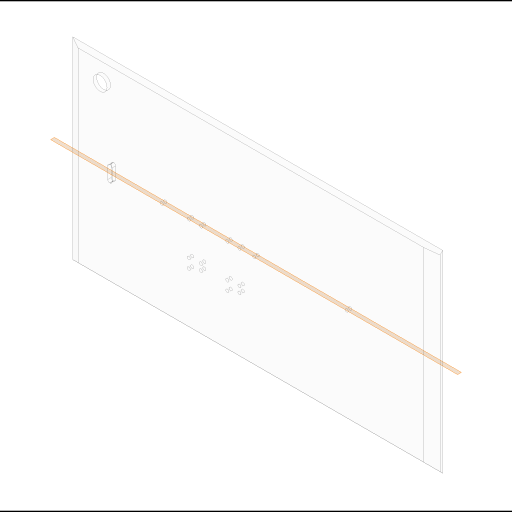
# Autodesk Inventor part: Wind Tunnel Test Section Bottom
Saved by Autodesk Inventor 2023 (Build 270158000, 158)
## iProperties
Created: 2022-03-05
Part Number: Wind Tunnel Test Section Bottom
Material: Polycarbonate, Clear
Document SubType Name: Modeling
Designer: kamer
Density: 1.2 g/cm^3
Appearance: Polycarbonate - Clear
Author: kamer
Autodesk Inventor part; units mm, degrees
ref_plane "YZ Plane" through (0, 0, 0) normal (1, 0, 0) x (0, 1, 0)
ref_plane "XY Plane" through (0, 0, 0) normal (0, 0, 1) x (1, 0, 0)
sketch "Sketch1" plane through (0, 0, 0) normal (0, 0, 1) x (1, 0, 0)
  line L0 (0, 0) -> (609.6, 0)
  line L1 (609.6, 0) -> (609.6, 317.881)
  line L2 (609.6, 317.881) -> (0, 317.881)
  line L3 (0, 317.881) -> (0, 0)
  dimension "d0" = 609.6
  dimension "d1" = 317.881
  constraints: 8 end point, 2 parallel, 1 horizontal, 1 perpendicular
  measures "d0" distance of L1.end L2.end
  measures "d1" distance of L0.end L1.end
extrude "Extrusion1" add sketch "Sketch1" along normal blind 5.7658
sketch "Sketch2" plane through (0, 317.881, 0) normal (0, 1, 0) x (1, 0, 0)
  line L0 (609.6, 0) -> (0, 0) projected
  line L1 (0, 0) -> (0, -5.7658) projected
  line L2 (609.6, -5.7658) -> (0, -5.7658) projected
  line L3 (609.6, 0) -> (609.6, -5.7658) projected
  line L4 (0, 0) -> (609.6, 0) projected
  line L5 (0, 0) -> (14.4594, -5.7658)
  line L6 (0, -5.7658) -> (609.6, -5.7658) projected
  line L7 (14.4594, -5.7658) -> (14.4594, 0)
  line L8 (14.4594, -5.7658) -> (20.2252, -5.7658) construction
  dimension "d4" = 21.74
  dimension "d5" = 90
  constraints: 6 end point, 2 point on line, 1 horizontal, 1 perpendicular
  measures "d4" angle of L5 L0
  measures "d5" angle of L8 L7
extrude "Extrusion2" cut sketch "Sketch2" against normal through all contours L5 L2 L1
sketch "Sketch3" plane through (609.6, 0, 0) normal (1, 0, 0) x (0, 0, -1)
  line L0 (0, 0) -> (0, 317.881) projected
  line L1 (0, 317.881) -> (-5.7658, 317.881) projected
  line L2 (-5.7658, 0) -> (-5.7658, 317.881) projected
  line L3 (0, 0) -> (-5.7658, 0) projected
  line L4 (0, 0) -> (-5.7658, 0) projected
  line L5 (0, 0) -> (-5.7658, 5.7658)
  line L6 (-5.7658, 0) -> (-5.7658, 317.881) projected
  line L7 (0, 0) -> (8.1541, 0) construction
  line L8 (0, 317.881) -> (-5.7658, 317.881) projected
  line L9 (0, 317.881) -> (-5.7658, 312.1152)
  line L10 (0, 317.881) -> (8.1541, 317.881) construction
  dimension "d8" = 135
  dimension "d9" = 135
  constraints: 8 end point, 2 equal length, 2 horizontal, 2 point on line
  measures "d8" angle of L7 L5
  measures "d9" angle of L9 L10
extrude "Extrusion3" cut sketch "Sketch3" against normal through all contours L3 L2 L5 | L9 L2 L1
ref_plane "Center Plane" through (0, 158.9405, 0) normal (0, 1, 0) x (-1, 0, 0)
sketch "Sketch4" plane through (0, 158.9405, 0) normal (0, 1, 0) x (-1, 0, 0)
  line L0 (-14.4594, 5.7658) -> (0, 0) projected
  line L1 (-609.6, 5.7658) -> (-14.4594, 5.7658) projected
  line L2 (-609.6, 0) -> (-609.6, 5.7658) projected
  line L3 (-609.6, 0) -> (0, 0) projected
  line L4 (-609.6, 5.7658) -> (-584.2, 5.7658) construction
  line L5 (-584.2, 5.7658) -> (-609.6, 4.4413)
  point P0 (0, 0)
  dimension "d13" = 25.4
  dimension "d14" = 2.985
  constraints: 4 end point, 2 point on line
  measures "d13" distance of L1.start L4.end
  measures "d14" angle of L4 L5
extrude "Extrusion4" cut sketch "Sketch4" against normal through all both and the other way through all contours L5 L2 L1
sketch "Sketch5" plane through (0, 0, 5.7658) normal (0, 0, 1) x (1, 0, 0)
  circle A0 centre (196.85, 158.9278) radius 2.5019
  line L0 (0, 317.881) -> (0, 0) projected
  line L1 (609.6, 317.881) -> (0, 317.881) projected
  circle A1 centre (260.35, 158.9405) radius 2.5019
  circle A2 centre (196.85, 103.5558) radius 2.5019
  circle A3 centre (260.35, 103.5685) radius 2.5019
  circle A4 centre (196.85, 88.3158) radius 2.5019
  circle A5 centre (260.35, 88.3285) radius 2.5019
  circle A6 centre (152.4, 158.9405) radius 2.5019
  circle A7 centre (304.8, 158.9405) radius 2.5019
  circle A8 centre (457.2, 158.9405) radius 2.5019
  line L2 (66.675, 145.7528) -> (67.325, 145.7528)
  line L3 (70.5, 148.9278) -> (70.5, 168.9278)
  line L4 (67.325, 172.1028) -> (66.675, 172.1028)
  line L5 (63.5, 168.9278) -> (63.5, 148.9278)
  line L6 (63.5, 145.7528) -> (70.5, 172.1028) construction
  line L7 (70.5, 145.7528) -> (63.5, 172.1028) construction
  arc A9 (70.5, 168.9278) -> (67.325, 172.1028) centre (67.325, 168.9278) ccw
  arc A10 (66.675, 172.1028) -> (63.5, 168.9278) centre (66.675, 168.9278) ccw
  arc A11 (63.5, 148.9278) -> (66.675, 145.7528) centre (66.675, 148.9278) ccw
  arc A12 (67.325, 145.7528) -> (70.5, 148.9278) centre (67.325, 148.9278) ccw
  point P0 (67, 158.9278)
  dimension "d17" = 196.85
  dimension "d18" = 158.9532
  dimension "d19" = 5.0038
  dimension "d20" = 63.5
  dimension "d21" = 5.0038
  dimension "d22" = 55.372
  dimension "d23" = 55.372
  dimension "d24" = 196.85
  dimension "d25" = 63.5
  dimension "d26" = 158.9405
  dimension "d27" = 5.0038
  dimension "d28" = 5.0038
  dimension "d29" = 15.24
  dimension "d30" = 15.24
  dimension "d31" = 5.0038
  dimension "d32" = 5.0038
  dimension "d33" = 63.5
  dimension "d34" = 196.85
  dimension "d35" = 152.4
  dimension "d36" = 5.0038
  dimension "d37" = 158.9405
  dimension "d38" = 304.8
  dimension "d39" = 5.0038
  dimension "d40" = 158.9405
  dimension "d41" = 457.2
  dimension "d42" = 158.9405
  dimension "d43" = 5.0038
  dimension "d44" = 3.175
  dimension "d45" = 7
  dimension "d46" = 20
  dimension "d47" = 158.9532
  dimension "d48" = 63.5
  constraints: 13 centre point, 12 end point, 8 point on circle, 8 point on line, 8 tangent, 3 equal radius, 2 midpoint, 2 parallel, 1 horizontal, 1 perpendicular
  measures "d17" distance from line of A0.centre L0
  measures "d18" distance from line of A0.centre L1
  measures "d19" diameter of A0
  measures "d20" distance of A1.centre A0.centre
  measures "d21" diameter of A1
  measures "d22" distance of A0.centre A2.centre
  measures "d23" distance of A3.centre A1.centre
  measures "d24" distance from line of L0 A2.centre
  measures "d25" distance of A2.centre A3.centre
  measures "d26" distance from line of L1 A1.centre
  measures "d27" diameter of A2
  measures "d28" diameter of A3
  measures "d29" distance of A4.centre A2.centre
  measures "d30" distance of A5.centre A3.centre
  measures "d31" diameter of A4
  measures "d32" diameter of A5
  measures "d33" distance of A4.centre A5.centre
  measures "d34" distance from line of L0 A4.centre
  measures "d35" distance from line of L0 A6.centre
  measures "d36" diameter of A6
  measures "d37" distance from line of A6.centre L1
  measures "d38" distance from line of L0 A7.centre
  measures "d39" diameter of A7
  measures "d40" distance from line of L1 A7.centre
  measures "d41" distance from line of L0 A8.centre
  measures "d42" distance from line of L1 A8.centre
  measures "d43" diameter of A8
  measures "d44" radius of A9
  measures "d45" distance between parallel lines of L3 L5
  measures "d46" distance of L3.start L3.end
  measures "d47" distance from line of L1 point (67, 158.928)
  measures "d48" distance between parallel lines of L0 L5
extrude "Extrusion5" cut sketch "Sketch5" against normal through all
sketch "Sketch6" plane through (0, 0, 5.7658) normal (0, 0, 1) x (1, 0, 0)
  circle A0 centre (50.8, 279.781) radius 11.43
  line L0 (609.6, 317.881) -> (0, 317.881) projected
  line L1 (0, 317.881) -> (0, 0) projected
  dimension "d51" = 38.1
  dimension "d52" = 50.8
  dimension "d53" = 22.86
  constraints: 1 centre point
  measures "d51" distance from line of L0 A0.centre
  measures "d52" distance from line of A0.centre L1
  measures "d53" diameter of A0
extrude "Extrusion6" cut sketch "Sketch6" against normal through all
sketch "Sketch7" plane through (0, 0, 5.7658) normal (0, 0, 1) x (1, 0, 0)
  circle A0 centre (216.85, 158.9278) radius 2.5
  circle A1 centre (196.85, 103.5558) radius 2.5019 construction
  circle A2 centre (196.85, 158.9278) radius 2.5019 construction
  line L0 (196.85, 103.5558) -> (196.85, 158.9278) construction
  line L1 (196.85, 158.9278) -> (216.85, 158.9278) construction
  line L2 (216.85, 158.9278) -> (216.85, 105.4278) construction
  circle A3 centre (216.85, 105.4278) radius 2.5
  circle A4 centre (196.85, 88.3158) radius 2.5019 construction
  line L3 (196.85, 103.5558) -> (196.85, 88.3158) construction
  line L4 (216.85, 95.4278) -> (216.85, 105.4278) construction
  circle A5 centre (216.85, 95.4278) radius 2.5
  line L5 (216.85, 158.9278) -> (280.35, 158.9278) construction
  line L6 (280.35, 158.9278) -> (280.35, 95.4278) construction
  line L7 (280.35, 95.4278) -> (280.35, 105.4278) construction
  circle A6 centre (280.35, 105.4278) radius 2.5
  circle A7 centre (280.35, 95.4278) radius 2.5
  circle A8 centre (280.35, 158.9278) radius 2.5
  circle A9 centre (260.35, 158.9405) radius 2.5019 projected
  point P0 (0, 0)
  dimension "d56" = 5
  dimension "d57" = 20
  dimension "d58" = 5
  dimension "d59" = 5
  dimension "d60" = 63.5
  dimension "d61" = 5
  dimension "d62" = 5
  dimension "d63" = 5
  dimension "d64" = 63.5
  dimension "d65" = 63.5
  dimension "d66" = 10
  dimension "d67" = 180
  dimension "d68" = 10
  constraints: 16 end point, 6 centre point, 5 coincident, 3 perpendicular, 1 horizontal, 1 point on line, 1 vertical
  measures "d56" diameter of A0
  measures "d57" distance between parallel lines of L0 L2
  measures "d58" diameter of A3
  measures "d59" diameter of A5
  measures "d60" distance of L1.end L5.end
  measures "d61" diameter of A6
  measures "d62" diameter of A7
  measures "d63" diameter of A8
  measures "d64" distance of L4.start L1.end
  measures "d65" distance of L5.end L6.end
  measures "d66" distance of L2.end L4.start
  measures "d67" angle of L4 L2
  measures "d68" distance of L7.end L6.end
extrude "Extrusion7" cut sketch "Sketch7" against normal through all contours A0 | A3 | A5 | A6 | A7 | A8
body "Solid1"
